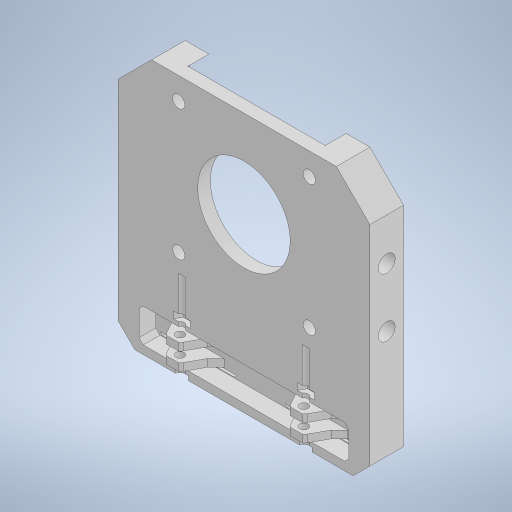
# Autodesk Inventor part: каретка_без_м
Saved by Autodesk Inventor 2023.1 (Build 271208000, 208)
## iProperties
Created: 2025-12-14
Part Number: каретка_без_м
Material: Типовые
Document SubType Name: Modeling
Designer: DELL
Density: 1 g/cm^3
Appearance: По умолчанию
Author: DELL
Autodesk Inventor part; units mm, degrees
ref_plane "YZ Plane" through (0, 0, 0) normal (1, 0, 0) x (0, 1, 0)
ref_plane "XZ Plane" through (0, 0, 0) normal (0, 1, 0) x (-1, 0, 0)
ref_plane "XY Plane" through (0, 0, 0) normal (0, 0, 1) x (1, 0, 0)
sketch "Эскиз1" plane through (0, 0, 0) normal (0, 0, 1) x (1, 0, 0)
  line L0 (16.9838, 20.6364) -> (20.6364, 16.9838) projected
  arc A0 (16.9838, 20.6364) -> (16.3474, 20.9) centre (16.3474, 20) ccw projected
  line L1 (-16.3474, 20.9) -> (16.3474, 20.9) projected
  arc A1 (-16.3474, 20.9) -> (-16.9838, 20.6364) centre (-16.3474, 20) ccw projected
  line L2 (-20.6364, 16.9838) -> (-16.9838, 20.6364) projected
  arc A2 (-20.6364, 16.9838) -> (-20.9, 16.3474) centre (-20, 16.3474) ccw projected
  line L3 (-20.9, -16.3474) -> (-20.9, 16.3474) projected
  arc A3 (-20.9, -16.3474) -> (-20.6364, -16.9838) centre (-20, -16.3474) ccw projected
  line L4 (-16.9838, -20.6364) -> (-20.6364, -16.9838) projected
  arc A4 (-16.9838, -20.6364) -> (-16.3474, -20.9) centre (-16.3474, -20) ccw projected
  line L5 (16.3474, -20.9) -> (-16.3474, -20.9) projected
  arc A5 (16.3474, -20.9) -> (16.9838, -20.6364) centre (16.3474, -20) ccw projected
  line L6 (20.6364, -16.9838) -> (16.9838, -20.6364) projected
  arc A6 (20.6364, -16.9838) -> (20.9, -16.3474) centre (20, -16.3474) ccw projected
  line L7 (20.9, 16.3474) -> (20.9, -16.3474) projected
  arc A7 (20.9, 16.3474) -> (20.6364, 16.9838) centre (20, 16.3474) ccw projected
  circle A8 centre (15.5574, -15.5574) radius 1.45 projected
  circle A9 centre (0, 0) radius 11 projected
  circle A10 centre (-15.5574, -15.5574) radius 1.45 projected
  circle A11 centre (-15.5574, 15.5574) radius 1.45 projected
  circle A12 centre (15.5574, 15.5574) radius 1.45 projected
  point P0 (0, 0)
extrude "Выдавливание1" add sketch "Эскиз1" along normal blind 3
sketch "Эскиз2" plane through (0, 0, 3) normal (0, 0, 1) x (1, 0, 0)
  line L0 (16.3474, 20.9) -> (-16.3474, 20.9) construction
  line L1 (-30, -20.9) -> (30, -20.9)
  line L2 (30, -20.9) -> (30, 20.9)
  line L3 (30, 20.9) -> (-30, 20.9)
  line L4 (-30, 20.9) -> (-30, -20.9)
  circle A0 centre (0, 0) radius 11 construction
  line L5 (-30, -20.9) -> (30, 20.9) construction
  line L6 (30, -20.9) -> (-30, 20.9) construction
  line L7 (-30, -20.9) -> (30, -20.9)
  line L8 (30, -20.9) -> (30, -40.9)
  line L9 (30, -40.9) -> (-30, -40.9)
  line L10 (-30, -40.9) -> (-30, -20.9)
  line L11 (-16.9838, 20.6364) -> (-20.6364, 16.9838) projected
  arc A1 (-20.6364, 16.9838) -> (-20.9, 16.3474) centre (-20, 16.3474) ccw projected
  line L12 (-20.9, 16.3474) -> (-20.9, -16.3474) projected
  arc A2 (-20.9, -16.3474) -> (-20.6364, -16.9838) centre (-20, -16.3474) ccw projected
  line L13 (-20.6364, -16.9838) -> (-16.9838, -20.6364) projected
  arc A3 (-16.9838, -20.6364) -> (-16.3474, -20.9) centre (-16.3474, -20) ccw projected
  line L14 (-16.3474, -20.9) -> (16.3474, -20.9) projected
  arc A4 (16.3474, -20.9) -> (16.9838, -20.6364) centre (16.3474, -20) ccw projected
  line L15 (16.9838, -20.6364) -> (20.6364, -16.9838) projected
  arc A5 (20.6364, -16.9838) -> (20.9, -16.3474) centre (20, -16.3474) ccw projected
  line L16 (20.9, -16.3474) -> (20.9, 16.3474) projected
  arc A6 (20.9, 16.3474) -> (20.6364, 16.9838) centre (20, 16.3474) ccw projected
  line L17 (20.6364, 16.9838) -> (16.9838, 20.6364) projected
  arc A7 (16.9838, 20.6364) -> (16.3474, 20.9) centre (16.3474, 20) ccw projected
  line L18 (16.3474, 20.9) -> (-16.3474, 20.9) projected
  arc A8 (-16.3474, 20.9) -> (-16.9838, 20.6364) centre (-16.3474, 20) ccw projected
  circle A9 centre (0, 0) radius 11 construction
  circle A10 centre (15.5574, 15.5574) radius 1.45 construction
  circle A11 centre (-15.5574, 15.5574) radius 1.45 construction
  circle A12 centre (-15.5574, -15.5574) radius 1.45 construction
  circle A13 centre (15.5574, -15.5574) radius 1.45 construction
  dimension "d4" = 60
  dimension "d5" = 60
  dimension "d6" = 20
  constraints: 20 end point, 4 parallel, 2 horizontal, 2 midpoint, 2 perpendicular
  measures "d4" distance of L3.end L2.end
  measures "d5" distance of L8.end L9.end
  measures "d6" distance of L7.end L8.end
extrude "Выдавливание2" add sketch "Эскиз2" against normal blind 8 contours L4 L3 A8 L11 A1 L12 A2 L13 A3 L1 | L1 L8 L9 L10 | A4 L15 A5 L16 A6 L17 A7 L3 L2 L1
sketch "Эскиз5" plane through (0, 0, 3) normal (0, 0, 1) x (1, 0, 0)
  line L0 (30, -40.9) -> (-30, -40.9) construction
  line L1 (0, -40.9) -> (0, 20.9) construction
  line L2 (16.3474, 20.9) -> (-16.3474, 20.9) construction
  line L3 (24, -30.9) -> (-24, -30.9)
  line L4 (-25, -31.9) -> (-25, -37.9)
  line L5 (-24, -38.9) -> (24, -38.9)
  line L6 (25, -37.9) -> (25, -31.9)
  line L7 (25, -30.9) -> (-25, -38.9) construction
  line L8 (-25, -30.9) -> (25, -38.9) construction
  line L9 (24, -30.9) -> (25, -31.9)
  line L10 (24, -38.9) -> (25, -37.9)
  line L11 (-25, -37.9) -> (-24, -38.9)
  line L12 (-24, -30.9) -> (-25, -31.9)
  point P0 (0, 0)
  point P1 (0, -34.9)
  dimension "d29" = 50
  dimension "d30" = 8
  dimension "d33" = 2
  dimension "d91" = 1
  dimension "d92" = 1
  dimension "d93" = 1
  dimension "d94" = 1
  dimension "d95" = 1
  dimension "d96" = 1
  dimension "d97" = 1
  dimension "d98" = 1
  constraints: 22 end point, 9 point on line, 4 midpoint, 2 parallel, 1 horizontal, 1 perpendicular
  measures "d29" distance of L8.end L7.end
  measures "d30" distance of L7.end L8.start
  measures "d33" distance between parallel lines of L0 L5
  measures "d91" distance of L3.start L7.start
  measures "d92" distance of L6.end L7.start
  measures "d93" distance of L5.end L8.end
  measures "d94" distance of L6.start L8.end
  measures "d95" distance of L4.end L7.end
  measures "d96" distance of L5.start L7.end
  measures "d97" distance of L3.end L8.start
  measures "d98" distance of L4.start L8.start
extrude "Выдавливание5" cut sketch "Эскиз5" against normal blind 4
ref_plane "РабПлоскость2" through (-23, -34.9, 3) normal (0, -1, 0) x (1, 0, 0)
sketch "Эскиз6" plane through (-23, -34.9, 3) normal (0, -1, 0) x (1, 0, 0)
  line L0 (-7, -8) -> (53, -8) construction
  line L1 (-7, -8) -> (53, -8) construction
  line L2 (53, -8) -> (53, -4) construction
  line L3 (53, -4) -> (-7, -4) construction
  line L4 (-7, -4) -> (-7, -8) construction
  line L5 (-7, -4) -> (8, -4) construction
  line L6 (8, -4) -> (8, -1.7967) construction
  line L7 (8, -1.7967) -> (-7, -1.7967) construction
  line L8 (-7, -1.7967) -> (-7, -4) construction
  circle A0 centre (8.2443, 0.4903) radius 1
  line L9 (-1, -4) -> (47, -4) projected
  line L10 (4.2443, -4) -> (12.2443, -4)
  line L11 (12.2443, -4) -> (12.2443, -2)
  line L12 (12.2443, -2) -> (4.2443, -2)
  line L13 (4.2443, -2) -> (4.2443, -4)
  line L14 (8.2443, 0.4903) -> (8.2443, -4) construction
  line L15 (4.2443, -2) -> (6.2303, 1.6011)
  line L16 (12.2443, -2) -> (10.2583, 1.6011)
  line L17 (4.2443, -2) -> (2.2406, -4)
  line L18 (4.2443, -2) -> (7.0754, -2) construction
  line L19 (12.2443, -2) -> (14.248, -4)
  arc A1 (10.2583, 1.6011) -> (6.2303, 1.6011) centre (8.2443, 0.4903) ccw construction
  arc A2 (6.7884, 2.2709) -> (9.7002, 2.2709) centre (8.2443, 0.4903) ccw
  line L20 (6.7884, 2.2709) -> (9.7002, 2.2709)
  point P0 (23, -3)
  point P1 (6.6526, -8)
  point P2 (8.2443, -2)
  point P3 (2.2406, -4)
  point P4 (6.2303, 1.6011)
  dimension "d36" = 4
  dimension "d37" = 15
  dimension "d40" = 2
  dimension "d41" = 8
  dimension "d42" = 2
  dimension "d61" = 4.4903
  constraints: 38 end point, 6 parallel, 5 horizontal, 5 point on circle, 4 perpendicular, 3 centre point, 3 point on line, 2 coincident, 2 midpoint, 1 equal length, 1 symmetric about line
  measures "d36" distance of L2.end L0.end
  measures "d37" distance of L7.end L6.end
  measures "d40" diameter of A0
  measures "d41" distance of L12.end L11.end
  measures "d42" distance of L11.end L10.end
  measures "d61" distance from line of L10 L14.start
extrude "Выдавливание6" add sketch "Эскиз6" along normal mid plane 6
extrude "Выдавливание7" cut sketch "Эскиз6" along normal mid plane 2.4
ref_plane "РабПлоскость3" through (0, -36.9, 3) normal (1, 0, 0) x (0, 0, -1)
sketch "Эскиз8" plane through (-23, -37.9, 3) normal (0, -1, 0) x (1, 0, 0)
  circle A0 centre (8.2443, 0.4903) radius 1 projected
  circle A1 centre (8.2443, 0.4903) radius 1 projected
  point P0 (23, -3)
extrude "Выдавливание8" cut sketch "Эскиз8" along normal blind 3 and the other way blind 18
sketch "Эскиз9" plane through (-30, -40.9, -5) normal (0, -1, 0) x (1, 0, 0)
  arc A0 (16.2443, 8.4903) -> (16.2443, 8.4903) centre (15.2443, 8.4903) ccw construction
  circle A1 centre (15.2443, 8.4903) radius 1.6
  point P0 (30, 5)
  dimension "d54" = 3.2
  constraints: 1 centre point, 1 coincident
  measures "d54" diameter of A1
extrude "Выдавливание9" cut sketch "Эскиз9" against normal blind 1
ref_plane "РабПлоскость4" through (-23, -29.9, -1) normal (0, -1, 0) x (1, 0, 0)
sketch "Эскиз10" plane through (-23, -29.9, -1) normal (0, -1, 0) x (1, 0, 0)
  circle A0 centre (8.2443, 4.4903) radius 1 construction
  line L0 (7.0906, 2.4897) -> (5.9349, 4.4891)
  line L1 (5.9349, 4.4891) -> (7.0886, 6.4897)
  line L2 (7.0886, 6.4897) -> (9.398, 6.4909)
  line L3 (9.398, 6.4909) -> (10.5537, 4.4915)
  line L4 (10.5537, 4.4915) -> (9.4, 2.4909)
  line L5 (9.4, 2.4909) -> (7.0906, 2.4897)
  point P0 (23, 1)
  dimension "d58" = 4
  constraints: 12 end point, 1 coincident, 13 other
  measures "d58" distance between parallel lines of L2 L5
extrude "Выдавливание10" cut sketch "Эскиз10" against normal blind 1.6
mirror "Зеркальное отражение1" about plane through (0, -36.9, 3) normal (1, 0, 0) of "Выдавливание6", "Выдавливание7", "Выдавливание8", "Выдавливание10", "Выдавливание9"
sketch "Эскиз11" plane through (0, 0, -5) normal (0, 0, -1) x (-1, 0, 0)
  line L0 (-8.752, -33.7) -> (-8.752, -31.9) construction
  line L1 (-8.752, -31.9) -> (-20.7594, -31.9) construction
  line L2 (-20.7594, -31.9) -> (-20.7594, -33.7) construction
  line L3 (-8.752, -33.7) -> (-20.7594, -33.7) construction
  line L4 (-20.7594, -36.1) -> (-8.752, -36.1) construction
  line L5 (-20.7594, -36.1) -> (-20.7594, -37.9) construction
  line L6 (-20.7594, -37.9) -> (-8.752, -37.9) construction
  line L7 (-8.752, -37.9) -> (-8.752, -36.1) construction
  line L8 (8.752, -36.1) -> (8.752, -37.9) construction
  line L9 (8.752, -37.9) -> (20.7594, -37.9) construction
  line L10 (20.7594, -37.9) -> (20.7594, -36.1) construction
  line L11 (20.7594, -36.1) -> (8.752, -36.1) construction
  line L12 (8.752, -33.7) -> (20.7594, -33.7) construction
  line L13 (20.7594, -33.7) -> (20.7594, -31.9) construction
  line L14 (20.7594, -31.9) -> (8.752, -31.9) construction
  line L15 (8.752, -31.9) -> (8.752, -33.7) construction
  line L16 (25, -37.9) -> (25, -31.9) projected
  line L17 (-24, -38.9) -> (24, -38.9) projected
  line L18 (-25, -31.9) -> (-25, -37.9) projected
  line L19 (24, -30.9) -> (-24, -30.9) projected
  line L20 (25, -31.9) -> (24, -30.9) projected
  line L21 (24, -38.9) -> (25, -37.9) projected
  line L22 (-25, -37.9) -> (-24, -38.9) projected
  line L23 (-24, -30.9) -> (-25, -31.9) projected
  point P0 (0, 0)
  point P1 (25, -38.9)
  point P2 (-25, -30.9)
  point P3 (-25, -38.9)
  point P4 (25, -30.9)
extrude "Выдавливание11" cut sketch "Эскиз11" against normal blind 3
sketch "Эскиз12" plane through (0, 0, -1) normal (0, 0, 1) x (1, 0, 0)
  line L0 (-12.3296, -33.8) -> (-17.3296, -33.8) construction
  line L1 (-12.3296, -36.1) -> (-17.3296, -36.1) construction
  line L2 (-12.3296, -33.8) -> (-17.3296, -33.8) construction
  line L3 (-12.3296, -36.1) -> (-17.3296, -36.1) construction
  line L4 (-17.3296, -33.8) -> (-12.3296, -36.1) construction
  line L5 (-5.8296, -38.1) -> (-23.8296, -38.1) construction
  line L6 (-23.8296, -38.1) -> (-23.8296, -31.8) construction
  line L7 (-23.8296, -31.8) -> (-5.8296, -31.8) construction
  line L8 (-5.8296, -31.8) -> (-5.8296, -38.1) construction
  line L9 (-5.8296, -38.1) -> (-23.8296, -31.8) construction
  line L10 (-23.8296, -38.1) -> (-5.8296, -31.8) construction
  line L11 (-23.8296, -31.8) -> (-5.8296, -31.8)
  line L12 (-5.8296, -31.8) -> (-5.8296, -31.7)
  line L13 (-6.3296, -31.2) -> (-23.3296, -31.2)
  line L14 (-23.8296, -31.7) -> (-23.8296, -31.8)
  line L15 (-23.8296, -38.1) -> (-5.8296, -38.1)
  line L16 (-5.8296, -38.1) -> (-5.8296, -38.2)
  line L17 (-6.3296, -38.7) -> (-23.3296, -38.7)
  line L18 (-23.8296, -38.2) -> (-23.8296, -38.1)
  line L19 (-5.8296, -31.7) -> (-6.3296, -31.2)
  line L20 (-23.3296, -31.2) -> (-23.8296, -31.7)
  line L21 (-23.8296, -38.2) -> (-23.3296, -38.7)
  line L22 (-5.8296, -38.2) -> (-6.3296, -38.7)
  point P0 (0, 0)
  point P1 (-14.8296, -34.95)
  point P2 (-5.8296, -31.2)
  point P3 (-23.8296, -31.2)
  point P4 (-5.8296, -38.7)
  point P5 (-23.8296, -38.7)
  dimension "d73" = 18
  dimension "d74" = 6.3
  dimension "d75" = 18
  dimension "d76" = 0.6
  dimension "d77" = 18
  dimension "d78" = 0.6
  constraints: 38 end point, 8 point on line, 6 parallel, 3 horizontal, 3 midpoint, 3 perpendicular
  measures "d73" distance of L6.end L7.end
  measures "d74" distance of L5.end L6.end
  measures "d75" distance of point (-23.83, -31.2) point (-5.83, -31.2)
  measures "d76" distance of point (-5.83, -31.2) L11.end
  measures "d77" distance of point (-5.83, -38.7) point (-23.83, -38.7)
  measures "d78" distance of L15.end point (-5.83, -38.7)
extrude "Выдавливание12" cut sketch "Эскиз12" against normal blind 3
mirror "Зеркальное отражение2" about plane through (0, -36.9, 3) normal (1, 0, 0) of "Выдавливание12"
chamfer "Фаска1" distance 4 angle 45 2 edges at (30, -40.9, -1) (-30, -40.9, -1)
chamfer "Фаска2" distance 8 angle 45 2 edges at (30, 20.9, -1) (-30, 20.9, -1)
sketch "Эскиз14" plane through (-30, -36.9, -5) normal (-1, 0, 0) x (0, 0, 1)
  line L0 (0, 49.8) -> (8, 49.8) construction
  line L1 (0, 0) -> (0, 49.8) construction
  line L2 (8, 0) -> (0, 0) construction
  line L3 (8, 49.8) -> (8, 0) construction
  line L4 (8, 49.8) -> (0, 49.8) projected
  line L5 (4, 49.8) -> (4, 0) construction
  line L6 (8, 0) -> (0, 0) projected
  circle A0 centre (4, 39.8) radius 2
  circle A1 centre (4, 25.8) radius 2
  dimension "d107" = 4
  dimension "d108" = 4
  dimension "d109" = 10
  dimension "d113" = 14
  constraints: 2 centre point, 2 end point, 2 midpoint, 2 point on line
  measures "d107" diameter of A0
  measures "d108" diameter of A1
  measures "d109" distance from line of L0 A0.centre
  measures "d113" distance of A1.centre A0.centre
extrude "Выдавливание13" cut sketch "Эскиз14" against normal blind 6
mirror "Зеркальное отражение3" about plane through (0, -36.9, 3) normal (1, 0, 0) of "Выдавливание13"
equation "\"d92\" = d91"
equation "\"d93\" = d91"
equation "\"d94\" = d93"
equation "\"d95\" = d91"
equation "\"d96\" = d95"
equation "\"d97\" = d91"
equation "\"d98\" = d97"
